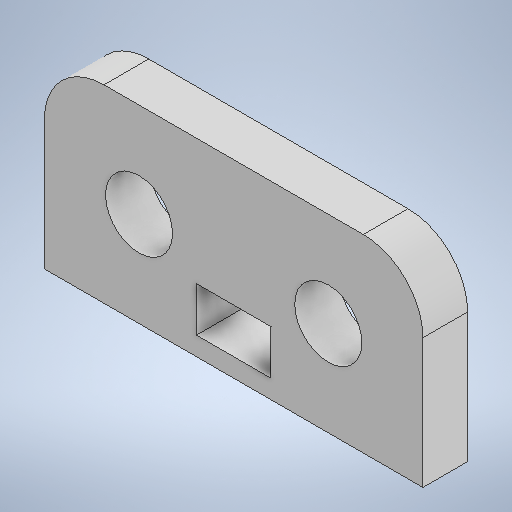
# Autodesk Inventor part: Moving Ramp Holder Base
Saved by Autodesk Inventor 2025.1 (Build 291241020, 241B)
## iProperties
Created: 2024-10-27
Part Number: Moving Ramp Holder Base
Material: Generic
Document SubType Name: Modeling
Designer: aly_g
Density: 1 g/cm^3
Appearance: Default
Author: aly_g
Autodesk Inventor part; units mm, degrees
ref_plane "YZ Plane" through (0, 0, 0) normal (1, 0, 0) x (0, 1, 0)
ref_plane "XZ Plane" through (0, 0, 0) normal (0, 1, 0) x (-1, 0, 0)
ref_plane "XY Plane" through (0, 0, 0) normal (0, 0, 1) x (1, 0, 0)
sketch "Sketch1" plane through (0, 0, 0) normal (0, 0, 1) x (1, 0, 0)
  line L0 (0, 0) -> (25.4, 0)
  line L1 (25.4, 0) -> (25.4, 12.7)
  line L2 (25.4, 12.7) -> (0, 12.7)
  line L3 (0, 12.7) -> (0, 0)
  dimension "d0" = 25.4
  dimension "d1" = 12.7
  constraints: 8 end point, 2 parallel, 1 horizontal, 1 perpendicular
  measures "d0" distance of L1.end L2.end
  measures "d1" distance of L0.start L2.end
extrude "Extrusion1" add sketch "Sketch1" along normal blind 3
fillet "Fillet1" radius 4 2 edges at (0, 12.7, 1.5) (25.4, 12.7, 1.5)
sketch "Sketch2" plane through (0, 0, 3) normal (0, 0, 1) x (1, 0, 0)
  line L0 (21.4, 12.7) -> (4, 12.7) projected
  line L1 (0, 8.7) -> (0, 0) projected
  line L2 (25.4, 0) -> (25.4, 8.7) projected
  line L3 (10.2, 4.25) -> (15.2, 4.25)
  line L4 (15.2, 4.25) -> (15.2, 1.25)
  line L5 (15.2, 1.25) -> (10.2, 1.25)
  line L6 (10.2, 1.25) -> (10.2, 4.25)
  line L7 (0, 0) -> (25.4, 0) projected
  point P0 (12.7, 12.7)
  point P1 (12.7, 4.25)
  point P2 (12.7, 0)
  point P3 (12.7, 1.25)
  point P4 (6.35, 6.35)
  point P5 (19.05, 6.35)
  dimension "d10" = 5
  dimension "d11" = 3
  dimension "d12" = 1.25
  dimension "d15" = 6.35
  dimension "d16" = 6.35
  dimension "d17" = 6.35
  constraints: 8 end point, 4 midpoint, 2 parallel, 1 horizontal, 1 horizontal alignment, 1 perpendicular, 1 vertical alignment
  measures "d10" distance of L4.end L5.end
  measures "d11" distance of L3.end L4.end
  measures "d12" distance of point (12.7, 0) point (12.7, 1.25)
  measures "d15" distance from line of L1 point (6.35, 6.35)
  measures "d16" distance from line of L0 point (6.35, 6.35)
  measures "d17" distance from line of L2 point (19.05, 6.35)
extrude "Extrusion2" cut sketch "Sketch2" against normal through all
hole "Hole1" at (19.05, 6.35, 3) at (6.35, 6.35, 3) direction (0, 0, -1) diameter 4.5 end through all clearance for "Flat Head Machine Screw" size "M4" standard "Ansi Metric M Profile"
body "Solid1"
